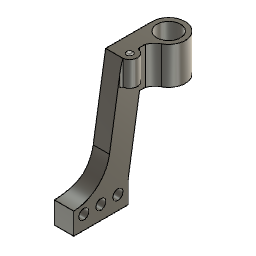
JRCNC0014 MIRROR v4 (Autodesk Fusion 360 design; units mm, degrees)
Autodesk Fusion 360 part; units mm, degrees
note: some values were not read from the file. Chosen so that the rebuilt part matches the saved one: how an offset face is resized. Set by a fixed rule: which sketch regions a step uses.
sketch "Sketch1" plane through (0, 0, 0) normal (0, 0, 1) x (1, 0, 0)
  circle A0 centre (0, 0) radius 7.625
  circle A1 centre (0, 0) radius 10.625
  line L0 (0, 0) -> (0, -7.5) construction
  line L1 (10.625, 0) -> (-10.625, 0)
  line L2 (-10.625, 0) -> (-10.625, -15)
  line L3 (-10.625, -15) -> (10.625, -15)
  line L4 (10.625, -15) -> (10.625, 0)
  line L5 (10.625, 0) -> (-10.625, -15) construction
  line L6 (-10.625, 0) -> (10.625, -15) construction
  line L7 (0, 0) -> (0, -15)
  point P0 (0, -7.5)
  dimension "d2" = 3
  dimension "d3" = 15.25
  dimension "d10" = 15
  constraint coincident A0.centre A1.centre
  constraint vertical L0
  constraint horizontal L1
  constraint perpendicular L1 L2
  constraint parallel L1 L3
  constraint parallel L2 L4
  constraint coincident A1 L1.start
  constraint coincident L5 P0
  constraint coincident L6 P0
  constraint coincident P0 L0.end
  constraint midpoint L3 L7.end
  measures "d2" distance of A0 A1
  measures "d3" diameter of A0
  measures "d10" distance of L1.end L2.end
extrude "Extrude1" add sketch "Sketch1" along normal blind 24 contours A0 A1 L1 L7 | A0 A1 L1 | A0 A1 L1 L7 | A1 L3 L4 L7 makes body 1
sketch "Sketch2" plane through (10.625, 0, 0) normal (1, 0, 0) x (0, -1, 0)
  line L0 (15, 0) -> (0, 0)
  line L1 (0, 0) -> (0, -24)
  line L2 (0, -24) -> (15, -24)
  line L3 (15, -24) -> (15, 0)
  line L4 (15, -24) -> (30, -24)
  line L5 (30, -24) -> (41.2502, 46)
  line L6 (41.2502, 46) -> (26.0578, 46)
  line L7 (26.0578, 46) -> (18.6568, -0.0492)
  line L8 (18.6568, -0.0492) -> (15, 0)
  point P0 (33.654, 46)
  dimension "d30" = 30
  dimension "d31" = 70
  dimension "d32" = 33.654
  dimension "d34" = 15
  constraint coincident L2.end L3.start
  constraint perpendicular L3 L4
  constraint perpendicular L3 L6
  constraint parallel L5 L7
  constraint coincident L0.start L3.end
  constraint midpoint L6 P0
  measures "d30" distance of L1 L4.end
  measures "d31" vertical distance of L1.end L6.end
  measures "d32" horizontal distance of L0.end P0
  measures "d34" distance of L5 L7
extrude "Extrude2" add sketch "Sketch2" against normal blind 10.5 contours L3 L4 L5 L6 L7 L8 bodies 1
sketch "Sketch3" plane through (10.625, 0, 0) normal (1, 0, 0) x (0, 1, 0)
  line L0 (0, 24) -> (-30, 24)
  line L1 (-61.0578, -46) -> (-26.0578, -46)
  line L2 (-26.0578, -46) -> (-26.0578, -60)
  line L3 (-26.0578, -60) -> (-61.0578, -60)
  line L4 (-61.0578, -60) -> (-61.0578, -46)
  line L5 (-15, 0) -> (0, 0)
  line L6 (0, 0) -> (0, 24)
  line L7 (-30, 24) -> (-41.2502, -46)
  line L8 (-41.2502, -46) -> (-26.0578, -46)
  line L9 (-26.0578, -46) -> (-18.6568, 0.0492)
  line L10 (-18.6568, 0.0492) -> (-15, 0)
  dimension "d26" = 14
  dimension "d27" = 35
  constraint horizontal L1
  constraint vertical L2
  constraint horizontal L3
  constraint vertical L4
  constraint coincident L1.end L2.start
  measures "d26" distance of L1.start L3.end
  measures "d27" distance of L2.end L3.end
extrude "Extrude3" add sketch "Sketch3" along normal blind 2 and the other way up to surface (10.5 mm away) contours L1 L2 L3 L4 L8 bodies 1
sketch "Sketch4" plane through (0.125, 0, 0) normal (-1, 0, 0) x (0, 1, 0)
  line L0 (-61.0578, 51) -> (-26.0578, 51) construction
  line L1 (-30, -24) -> (-15, -24)
  line L2 (-15, -24) -> (-15, 0)
  line L3 (-15, 0) -> (-18.6568, -0.0492)
  line L4 (-18.6568, -0.0492) -> (-26.0578, 46)
  line L5 (-26.0578, 46) -> (-26.0578, 60)
  line L6 (-26.0578, 60) -> (-61.0578, 60)
  line L7 (-61.0578, 60) -> (-61.0578, 46)
  line L8 (-61.0578, 46) -> (-41.2502, 46)
  line L9 (-41.2502, 46) -> (-30, -24)
  point P0 (-54.5578, 51)
  point P1 (-43.5578, 51)
  point P2 (-32.5578, 51)
  dimension "d20" = 11
  dimension "d21" = 11
  dimension "d44" = 5
  constraint coincident L0 P0
  constraint coincident L0 P2
  constraint horizontal L0
  constraint coincident L0 P1
  constraint coincident L0.start L7
  constraint midpoint L0 P1
  constraint coincident L0.end L5
  measures "d20" distance of P0 P1
  measures "d21" distance of P1 P2
  measures "d44" distance of L0 L8
hole "Hole1" at (0.125, -32.5578, -51) at (0.125, -43.5578, -51) at (0.125, -54.5578, -51) direction (1, 0, 0) diameter 3.4 depth 60 tip angle 180 counterbore diameter 6.5 counterbore depth 7 bodies 1
fillet "Fillet1" radius 9.5 1 edges at (0, -10.625, 12) on bodies 1
fillet "Fillet1" radius 24 2 edges at (5.375, -41.2502, -46) (10.625, -33.654, -46) on bodies 1
mirror "Mirror2" about plane through (12.625, 0, 0) normal (1, 0, 0) of bodies 1 makes body 2
sketch "Sketch5" plane through (0, 0, 24) normal (0, 0, 1) x (-1, 0, 0)
  circle A0 centre (-25.25, 0) radius 7.625
  arc A1 (-30.0103, 9.499) -> (-14.625, 0) centre (-25.25, 0) ccw
  line L0 (-14.625, 0) -> (-14.625, 30)
  line L1 (-14.625, 30) -> (-25.125, 30)
  line L2 (-25.125, 30) -> (-25.125, 15)
  line L3 (-25.125, 15) -> (-25.25, 15)
  arc A2 (-30.0103, 9.499) -> (-25.25, 15) centre (-34.2665, 17.9922) ccw
  circle A3 centre (-25.125, 25) radius 5
  dimension "d51" = 25
  constraint coincident L2 A3.centre
  constraint tangent L1 A3
  measures "d51" vertical distance of A0.centre A3.centre
extrude "Extrude4" add sketch "Sketch5" against normal blind 16 contours L2 A3 | L2 A3 bodies 2
hole "Hole2" at (25.125, -25, 24) direction (0, 0, -1) diameter 3.823 depth 13 tip angle 180 bodies 2
thread "Thread1" "ANSI Unified Screw Threads 0.19(#10) 10-32 UNF 2B" major diameter 4.826 minor diameter 4.064 pitch 0.7937 angle 60 resizes the face on face at (25.3153, -26.902, 15.3333) on bodies 2
fillet "Fillet2" radius 1.5 2 edges at (25.125, -30, 16) (25.125, -20, 16) on bodies 2
hidden bodies 1
equation "d32 = 45 mm - 11.346 mm"
